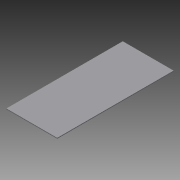
# Autodesk Inventor part: rueckteil
Saved by Autodesk Inventor 2013 (Build 170138000, 138)
## iProperties
Created: 2014-03-27
Part Number: rueckteil
Material: Generic
Document SubType Name: Modeling
Designer: hhanff
Density: 1 g/cm^3
Author: hhanff
Autodesk Inventor part; units mm, degrees
ref_plane "YZ Plane" through (0, 0, 0) normal (1, 0, 0) x (0, 1, 0)
ref_plane "XZ Plane" through (0, 0, 0) normal (0, 1, 0) x (-1, 0, 0)
ref_plane "XY Plane" through (0, 0, 0) normal (0, 0, 1) x (1, 0, 0)
sketch "Sketch1" plane through (0, 0, 0) normal (0, 0, 1) x (1, 0, 0)
  line L0 (0, 0) -> (520, 0)
  line L1 (520, 0) -> (520, 1190)
  line L2 (520, 1190) -> (0, 1190)
  line L3 (0, 1190) -> (0, 0)
  dimension "d0" = 1190
  dimension "d1" = 520
  constraints: 8 end point, 2 parallel, 1 horizontal, 1 perpendicular
  measures "d0" distance of L2.end L0.start
  measures "d1" distance of L0.start L0.end
extrude "Extrusion1" add sketch "Sketch1" along normal blind 8
body "Solid1"
